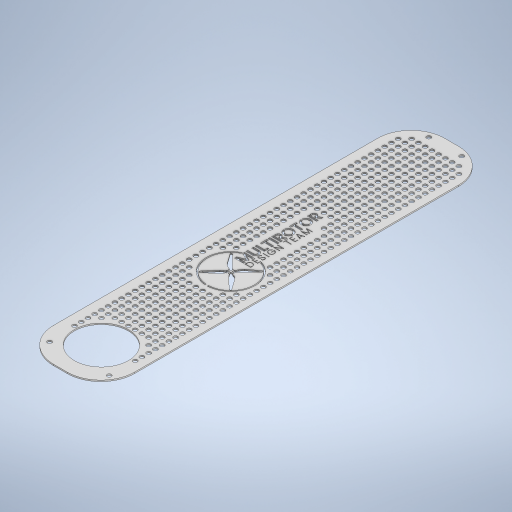
# Autodesk Inventor part: Ground station cover II
Saved by Autodesk Inventor 2023 (Build 270158000, 158)
## iProperties
Created: 2023-04-06
Part Number: Ground station cover II
Material: Generic
Document SubType Name: Modeling
Designer: mikep
Density: 1 g/cm^3
Appearance: Default
Author: mikep
Autodesk Inventor part; units mm, degrees
ref_plane "YZ Plane" through (0, 0, 0) normal (1, 0, 0) x (0, 1, 0)
ref_plane "XZ Plane" through (0, 0, 0) normal (0, 1, 0) x (-1, 0, 0)
ref_plane "XY Plane" through (0, 0, 0) normal (0, 0, 1) x (1, 0, 0)
sketch "Sketch1" plane through (0, 0, 0) normal (0, 1, 0) x (-1, 0, 0)
  line L0 (76.2, 0) -> (76.2, -342.9)
  line L1 (76.2, -342.9) -> (0, -342.9)
  line L2 (0, -342.9) -> (0, 0)
  line L3 (76.2, 0) -> (76.2, 25.4266)
  line L4 (76.2, 25.4266) -> (0, 25.4266)
  line L5 (0, 25.4266) -> (0, 0)
  constraints: 12 end point, 1 collinear, 1 parallel, 1 perpendicular, 1 vertical
extrude "Extrusion1" add sketch "Sketch1" along normal blind 1.27
sketch "Sketch4" plane through (0, 1.27, 0) normal (0, 1, 0) x (1, 0, 0)
  line L0 (-80.9566, 247.2278) -> (206.594, 247.2278)
  line L1 (206.594, 247.2278) -> (206.594, 87.4775)
  line L2 (206.594, 87.4775) -> (-80.9566, 87.4775)
  line L3 (-80.9566, 87.4775) -> (-80.9566, 247.2278)
  line L4 (-41.6156, 195.7662) -> (-41.6156, 195.7662)
  line L5 (-41.6156, 189.984) -> (-41.6156, 189.984)
  line L6 (-45.9155, 181.21) -> (-37.2389, 181.21)
  line L7 (-37.2389, 181.21) -> (-37.2389, 182.9014)
  line L8 (-37.2389, 182.9014) -> (-40.6526, 182.9014)
  line L9 (-40.6526, 183.7206) -> (-37.2389, 185.6718)
  line L10 (-37.2389, 185.6718) -> (-37.2389, 187.5783)
  line L11 (-37.2389, 187.5783) -> (-40.7469, 185.5482)
  arc A0 (-40.7469, 185.5482) -> (-45.5892, 186.0256) centre (-43.2468, 184.9881) ccw
  arc A1 (-45.5892, 186.0256) -> (-45.9155, 184.4827) centre (-42.1055, 184.4827) ccw
  line L12 (-44.4996, 182.9014) -> (-41.931, 182.9014)
  line L13 (-41.931, 183.7206) -> (-41.931, 184.5099)
  line L14 (-44.4996, 183.7206) -> (-44.4996, 184.5099)
  arc A2 (-41.931, 184.5099) -> (-44.4996, 184.5099) centre (-43.2153, 184.5099) ccw
  line L15 (-44.4996, 182.9014) -> (-45.9155, 182.9014)
  line L16 (-41.931, 182.9014) -> (-40.6526, 182.9014)
  line L17 (-40.6526, 183.7206) -> (-41.931, 183.7206)
  line L18 (-44.4996, 183.7206) -> (-45.9155, 183.7206)
  line L19 (-45.9155, 181.21) -> (-45.9155, 182.9014)
  line L20 (-45.9155, 183.7206) -> (-45.9155, 184.4827)
  line L21 (-44.4639, 192.4254) -> (-46.0536, 192.4254)
  line L22 (-44.4639, 193.4122) -> (-46.0419, 193.4122)
  line L23 (-38.7674, 192.4254) -> (-37.1776, 192.4254)
  line L24 (-37.1894, 193.4122) -> (-38.7674, 193.4122)
  arc A3 (-41.6156, 189.984) -> (-38.7674, 192.4254) centre (-41.6156, 192.8661) ccw
  arc A4 (-38.7674, 193.4122) -> (-41.6156, 195.7662) centre (-41.6156, 192.8661) ccw
  arc A5 (-37.1894, 193.4122) -> (-46.0419, 193.4122) centre (-41.6156, 192.8661) ccw
  arc A6 (-46.0536, 192.4254) -> (-37.1776, 192.4254) centre (-41.6156, 192.8661) ccw
  arc A7 (-44.4639, 192.4254) -> (-41.6156, 189.984) centre (-41.6156, 192.8661) ccw
  arc A8 (-41.6156, 195.7662) -> (-44.4639, 193.4122) centre (-41.6156, 192.8661) ccw
  point P0 (0, 0)
  point P1 (-41.6156, 195.7662)
  constraints: 42 end point, 18 point on circle, 9 centre point, 9 tangent, 8 perpendicular, 6 point on line, 4 horizontal, 3 concentric, 3 vertical, 2 parallel, 2 other
sketch "Sketch5" plane through (0, 1.27, 0) normal (0, 1, 0) x (1, 0, 0)
  line L0 (-45.9155, 146.2008) -> (-37.3157, 146.2008)
  line L1 (-37.3157, 146.2008) -> (-37.3157, 147.9554)
  line L2 (-37.3157, 147.9554) -> (-42.8395, 147.9554)
  line L3 (-42.8395, 147.9554) -> (-37.3157, 150.2733)
  line L4 (-37.3157, 150.2733) -> (-37.3157, 151.6596)
  line L5 (-37.3157, 151.6596) -> (-42.8395, 153.9342)
  line L6 (-42.8395, 153.9342) -> (-37.3157, 153.9342)
  line L7 (-37.3157, 153.9342) -> (-37.3157, 155.6671)
  line L8 (-37.3157, 155.6671) -> (-45.9155, 155.6671)
  line L9 (-45.9155, 155.6671) -> (-45.9155, 153.7609)
  line L10 (-45.9155, 153.7609) -> (-39.5036, 150.9664)
  line L11 (-39.5036, 150.9664) -> (-45.9155, 148.2759)
  line L12 (-45.9155, 148.2759) -> (-45.9155, 146.2008)
  line L13 (-45.9155, 157.0446) -> (-40.7133, 157.0446)
  arc A0 (-40.7133, 157.0446) -> (-40.7133, 164.1529) centre (-40.7133, 160.5987) ccw
  line L14 (-40.7133, 164.1529) -> (-45.9155, 164.1529)
  line L15 (-45.9155, 164.1529) -> (-45.9155, 162.4414)
  line L16 (-45.9155, 162.4414) -> (-40.4687, 162.4414)
  arc A1 (-40.4687, 158.8303) -> (-40.4687, 162.4414) centre (-40.4687, 160.6359) ccw
  line L17 (-40.4687, 158.8303) -> (-45.9155, 158.8303)
  line L18 (-45.9155, 158.8303) -> (-45.9155, 157.0446)
  line L19 (-45.9155, 165.5688) -> (-37.3157, 165.5688)
  line L20 (-37.3157, 165.5688) -> (-37.3157, 170.1637)
  line L21 (-37.3157, 170.1637) -> (-38.7004, 170.1637)
  line L22 (-41.8983, 212.0398) -> (-41.3637, 212.0398)
  line L23 (-41.3637, 206.7132) -> (-41.8983, 206.7132)
  line L24 (-45.9155, 197.9622) -> (-45.9155, 204.2278)
  line L25 (-45.9155, 204.2278) -> (-44.5825, 204.2278)
  line L26 (-44.5825, 204.2278) -> (-44.5825, 202.014)
  line L27 (-44.5825, 202.014) -> (-37.2602, 202.014)
  line L28 (-37.2602, 202.014) -> (-37.2602, 200.2387)
  line L29 (-37.2602, 200.2387) -> (-44.5825, 200.2387)
  line L30 (-44.5825, 200.2387) -> (-44.5825, 197.9622)
  line L31 (-44.5825, 197.9622) -> (-45.9155, 197.9622)
  line L32 (-45.9155, 165.5688) -> (-45.9155, 167.334)
  line L33 (-45.9155, 167.334) -> (-38.7004, 167.334)
  line L34 (-38.7004, 167.334) -> (-38.7004, 170.1637)
  line L35 (-45.9155, 170.5777) -> (-45.9155, 176.9008)
  line L36 (-45.9155, 176.9008) -> (-44.5825, 176.9008)
  line L37 (-44.5825, 176.9008) -> (-44.5825, 174.6319)
  line L38 (-44.5825, 174.6319) -> (-37.2602, 174.6319)
  line L39 (-37.2602, 174.6319) -> (-37.2602, 172.8987)
  line L40 (-37.2602, 172.8987) -> (-44.5825, 172.8987)
  line L41 (-44.5825, 172.8987) -> (-44.5825, 170.5777)
  line L42 (-44.5825, 170.5777) -> (-45.9155, 170.5777)
  line L43 (-45.9155, 177.9182) -> (-37.2602, 177.9182)
  line L44 (-37.2602, 177.9182) -> (-37.2602, 179.7056)
  line L45 (-37.2602, 179.7056) -> (-45.9155, 179.7056)
  line L46 (-45.9155, 179.7056) -> (-45.9155, 177.9182)
  line L47 (-45.9123, 214.8446) -> (-37.2357, 214.8446)
  line L48 (-37.2357, 214.8446) -> (-37.2357, 216.536)
  line L49 (-37.2357, 216.536) -> (-40.6494, 216.536)
  line L50 (-40.6494, 217.3525) -> (-40.6494, 217.3552)
  line L51 (-40.6494, 217.3552) -> (-37.2357, 219.3064)
  line L52 (-37.2357, 219.3064) -> (-37.2357, 221.2129)
  line L53 (-37.2357, 221.2129) -> (-40.7436, 219.1829)
  arc A2 (-40.7436, 219.1829) -> (-45.5859, 219.6602) centre (-43.2435, 218.6227) ccw
  arc A3 (-45.5859, 219.6602) -> (-45.9123, 218.1173) centre (-42.1022, 218.1173) ccw
  line L54 (-44.4963, 216.536) -> (-41.9277, 216.536)
  line L55 (-41.9277, 217.3525) -> (-41.9277, 218.1446)
  line L56 (-44.4963, 217.1678) -> (-44.4963, 218.1446)
  arc A4 (-41.9277, 218.1446) -> (-44.4963, 218.1446) centre (-43.212, 218.1446) ccw
  line L57 (-36.1361, 146.2008) -> (-30.6109, 146.2008)
  arc A5 (-30.6109, 148.0046) -> (-36.1361, 148.0046) centre (-33.3735, 148.0046) ccw
  line L58 (-35.7015, 146.7358) -> (-31.0051, 146.7358)
  arc A6 (-31.0051, 147.9604) -> (-35.7015, 147.9604) centre (-33.3533, 147.9604) ccw
  line L59 (-36.2043, 155.6671) -> (-36.2043, 152.7969)
  line L60 (-36.2043, 152.7969) -> (-30.6109, 152.7969)
  line L61 (-30.6109, 152.7969) -> (-30.6109, 155.6671)
  line L62 (-30.6109, 155.6671) -> (-31.0051, 155.6671)
  line L63 (-31.0051, 155.6671) -> (-31.0051, 153.3096)
  line L64 (-31.0051, 153.3096) -> (-33.1818, 153.3096)
  line L65 (-33.1818, 153.3096) -> (-33.1818, 155.4455)
  line L66 (-33.1818, 155.4455) -> (-33.6491, 155.4455)
  line L67 (-33.6491, 155.4455) -> (-33.6491, 153.3096)
  line L68 (-33.6491, 153.3096) -> (-35.7015, 153.3096)
  line L69 (-35.7015, 153.3096) -> (-35.7015, 155.6671)
  line L70 (-35.7015, 155.6671) -> (-36.2043, 155.6671)
  arc A7 (-34.9009, 160.6161) -> (-34.4089, 158.0946) centre (-34.5795, 159.3701) ccw
  arc A8 (-34.9009, 161.1543) -> (-34.4866, 157.5247) centre (-34.573, 159.3533) ccw
  arc A9 (-34.4866, 157.5247) -> (-33.5978, 158.2134) centre (-34.5328, 158.5023) ccw
  arc A10 (-34.4089, 158.0946) -> (-33.9237, 158.5805) centre (-34.6273, 158.7979) ccw
  line L71 (-33.9237, 158.5805) -> (-33.4038, 160.2634)
  line L72 (-33.5978, 158.2134) -> (-33.0272, 160.0606)
  arc A11 (-31.1407, 160.1849) -> (-33.0272, 160.0606) centre (-32.0602, 159.7619) ccw
  arc A12 (-30.6757, 160.2518) -> (-33.4038, 160.2634) centre (-32.0415, 159.8426) ccw
  arc A13 (-31.1407, 158.6615) -> (-31.1407, 160.1849) centre (-32.7961, 159.4232) ccw
  arc A14 (-32.0271, 158.1529) -> (-31.1407, 158.6615) centre (-31.9411, 159.0298) ccw
  arc A15 (-30.8736, 158.0903) -> (-30.6757, 160.2518) centre (-33.4619, 159.417) ccw
  arc A16 (-32.0271, 157.6019) -> (-30.8736, 158.0903) centre (-31.7422, 158.5356) ccw
  line L73 (-32.0271, 157.6019) -> (-32.0271, 158.1529)
  line L74 (-36.2043, 163.2972) -> (-30.5655, 163.2972)
  line L75 (-30.5655, 163.2972) -> (-30.5655, 163.8154)
  line L76 (-30.5655, 163.8154) -> (-36.2043, 163.8154)
  line L77 (-36.2043, 163.8154) -> (-36.2043, 163.2972)
  line L78 (-34.6103, 170.4888) -> (-34.6103, 171.0587)
  arc A17 (-34.6103, 170.4888) -> (-34.6103, 166.6847) centre (-33.6858, 168.5867) ccw
  arc A18 (-34.6103, 171.0587) -> (-34.6103, 166.0747) centre (-33.5706, 168.5667) ccw
  arc A19 (-34.6103, 166.6847) -> (-32.1267, 166.6847) centre (-33.3685, 169.1007) ccw
  arc A20 (-34.6103, 166.0747) -> (-32.1447, 166.0853) centre (-33.39, 168.9994) ccw
  arc A21 (-32.1267, 166.6847) -> (-32.1267, 170.4888) centre (-33.1517, 168.5867) ccw
  arc A22 (-32.1447, 166.0853) -> (-32.1447, 171.1174) centre (-33.3594, 168.6014) ccw
  line L79 (-32.1447, 166.0853) -> (-32.1447, 171.1174) construction
  line L80 (-32.1447, 166.0853) -> (-27.1125, 166.0853) construction
  arc A23 (-32.1267, 170.4888) -> (-33.0883, 170.6871) centre (-32.9388, 168.9819) ccw
  arc A24 (-32.1447, 171.1174) -> (-32.9486, 171.3013) centre (-32.9486, 169.4522) ccw
  line L81 (-33.0883, 170.6871) -> (-33.0883, 168.3488)
  line L82 (-33.0883, 168.3488) -> (-33.5713, 168.3488)
  line L83 (-33.5713, 168.3488) -> (-33.5713, 171.3013)
  line L84 (-33.5713, 171.3013) -> (-32.9486, 171.3013)
  line L85 (-30.5851, 173.2809) -> (-36.2043, 173.2809)
  line L86 (-36.2043, 173.2809) -> (-36.2043, 173.8147)
  line L87 (-36.2043, 173.8147) -> (-31.5027, 176.9008)
  line L88 (-31.5027, 176.9008) -> (-36.2043, 176.9008)
  line L89 (-36.2043, 176.9008) -> (-36.2043, 177.5031)
  line L90 (-36.2043, 177.5031) -> (-30.5851, 177.5031)
  line L91 (-30.5851, 177.5031) -> (-30.5851, 176.9008)
  line L92 (-30.5851, 176.9008) -> (-35.2868, 173.8147)
  line L93 (-35.2868, 173.8147) -> (-30.5851, 173.8147)
  line L94 (-30.5851, 173.8147) -> (-30.5851, 173.2809)
  line L95 (-36.2043, 182.4231) -> (-36.2043, 186.111)
  line L96 (-36.2043, 186.111) -> (-35.7015, 186.111)
  line L97 (-35.7015, 186.111) -> (-35.7015, 184.5808)
  line L98 (-35.7015, 184.5808) -> (-30.5851, 184.5808)
  line L99 (-30.5851, 184.5808) -> (-30.5851, 184.0076)
  line L100 (-30.5851, 184.0076) -> (-35.7015, 184.0076)
  line L101 (-35.7015, 184.0076) -> (-35.7015, 182.4231)
  line L102 (-35.7015, 182.4231) -> (-36.2043, 182.4231)
  line L103 (-36.2043, 187.9758) -> (-36.2043, 190.8754)
  line L104 (-36.2043, 190.8754) -> (-35.7464, 190.8754)
  line L105 (-35.7464, 190.8754) -> (-35.7464, 188.5016)
  line L106 (-35.7464, 188.5016) -> (-33.6172, 188.5016)
  line L107 (-33.6172, 188.5016) -> (-33.6172, 190.6504)
  line L108 (-33.6172, 190.6504) -> (-33.1818, 190.6504)
  line L109 (-33.1818, 190.6504) -> (-33.2075, 188.4955)
  line L110 (-33.2075, 188.4955) -> (-31.0568, 188.4699)
  line L111 (-31.0568, 188.4699) -> (-31.0286, 190.8383)
  line L112 (-31.0286, 190.8383) -> (-30.5851, 190.833)
  line L113 (-30.5851, 190.833) -> (-30.6192, 187.9758)
  line L114 (-30.6192, 187.9758) -> (-36.2043, 187.9758)
  line L115 (-36.0981, 194.6003) -> (-36.0981, 195.1894)
  line L116 (-30.5379, 197.1874) -> (-30.5379, 196.6332)
  line L117 (-30.5379, 196.6332) -> (-31.8644, 196.1565)
  line L118 (-31.8644, 193.5948) -> (-30.5379, 193.1069)
  line L119 (-30.5379, 193.1069) -> (-30.5379, 192.5551)
  line L120 (-30.6192, 199.1004) -> (-36.0958, 199.1004)
  line L121 (-36.0958, 199.1004) -> (-36.0958, 199.6747)
  line L122 (-36.0958, 199.6747) -> (-31.3653, 201.8102)
  line L123 (-31.3653, 201.8102) -> (-36.0958, 203.9571)
  line L124 (-36.0958, 203.9571) -> (-36.0958, 204.5166)
  line L125 (-36.0958, 204.5166) -> (-30.6192, 204.5166)
  line L126 (-30.6192, 204.5166) -> (-30.6192, 204.0028)
  line L127 (-30.6192, 204.0028) -> (-35.0644, 204.0028)
  line L128 (-35.0644, 204.0028) -> (-30.6192, 201.9853)
  line L129 (-30.6192, 201.9853) -> (-30.6192, 201.6879)
  line L130 (-30.6192, 201.6879) -> (-34.9638, 199.6747)
  line L131 (-34.9638, 199.6747) -> (-30.6192, 199.6747)
  line L132 (-30.6192, 199.6747) -> (-30.6192, 199.1004)
  line L133 (-29.8128, 154.4415) -> (-29.8128, 155.5845)
  line L134 (-46.6367, 153.1669) -> (-46.6367, 154.3802)
  arc A25 (-37.3019, 131.531) -> (-38.3544, 129.2661) centre (-33.6753, 128.4687) ccw
  arc A26 (-39.931, 126.4634) -> (-38.3544, 129.2661) centre (-43.0594, 130.0679) ccw
  line L135 (-39.931, 126.4634) -> (-51.2653, 117.782)
  arc A27 (-51.6556, 119.3522) -> (-51.2653, 117.782) centre (-50.6262, 118.7744) ccw
  arc A28 (-50.7672, 120.6762) -> (-51.6556, 119.3522) centre (-42.9118, 114.4448) ccw
  line L136 (-50.7672, 120.6762) -> (-43.0339, 129.1527)
  arc A29 (-40.9214, 131.0009) -> (-43.0339, 129.1527) centre (-33.7965, 120.7253) ccw
  arc A30 (-40.9214, 131.0009) -> (-38.9896, 132.5554) centre (-50.8331, 145.2957) ccw
  arc A31 (-35.5046, 136.0705) -> (-35.3221, 136.4134) centre (-35.9841, 136.5458) ccw
  arc A32 (-34.5137, 138.6581) -> (-35.3221, 136.4134) centre (-27.4046, 134.8301) ccw
  arc A33 (-31.9411, 142.1183) -> (-34.5137, 138.6581) centre (-21.4115, 131.6031) ccw
  line L137 (-31.9411, 142.1183) -> (-22.0341, 149.4341)
  arc A34 (-21.5184, 147.9604) -> (-22.0341, 149.4341) centre (-22.6014, 148.4085) ccw
  arc A35 (-22.1375, 147.004) -> (-21.5184, 147.9604) centre (-24.4242, 149.1628) ccw
  line L138 (-22.1375, 147.004) -> (-32.1455, 136.4032)
  arc A36 (-32.6979, 135.9774) -> (-32.1455, 136.4032) centre (-33.7632, 137.9304) ccw
  arc A37 (-32.6979, 135.9774) -> (-34.232, 134.8088) centre (-29.6411, 130.3732) ccw
  arc A38 (-34.7465, 133.0816) -> (-31.7342, 131.6031) centre (-30.9458, 137.0173) ccw
  arc A39 (-30.3913, 131.0009) -> (-31.7342, 131.6031) centre (-32.1221, 128.9395) ccw
  arc A40 (-27.8576, 128.297) -> (-30.3913, 131.0009) centre (-40.3881, 119.0944) ccw
  line L139 (-27.8939, 128.3463) -> (-21.0506, 118.672)
  arc A41 (-22.9089, 118.3552) -> (-21.0506, 118.672) centre (-22.1356, 119.4277) ccw
  arc A42 (-24.0971, 119.3522) -> (-22.9089, 118.3552) centre (-16.7176, 126.9409) ccw
  line L140 (-24.0971, 119.3522) -> (-33.3887, 128.4687)
  arc A43 (-35.1974, 130.7141) -> (-33.3887, 128.4687) centre (-24.7254, 137.2984) ccw
  line L141 (-35.1974, 130.7141) -> (-36.0908, 131.7691)
  line L142 (-38.4118, 134.2018) -> (-38.9896, 134.8301)
  arc A44 (-37.8105, 136.1187) -> (-38.8384, 137.4254) centre (-53.9232, 124.5022) ccw
  line L143 (-38.8384, 137.4254) -> (-49.6093, 148.2759)
  arc A45 (-49.6093, 148.2759) -> (-50.5164, 148.9551) centre (-52.3671, 145.5384) ccw
  arc A46 (-50.5164, 148.9551) -> (-52.0337, 148.4508) centre (-50.9672, 147.7767) ccw
  line L144 (-52.0337, 148.4508) -> (-45.145, 138.6581)
  arc A47 (-45.145, 138.6581) -> (-42.0297, 136.1187) centre (-39.0672, 142.9336) ccw
  arc A48 (-42.0297, 136.1187) -> (-38.9896, 134.8301) centre (29.7401, 301.2179) ccw
  line L145 (-35.7015, 147.1027) -> (-36.1361, 147.1027)
  line L146 (-35.7015, 147.5439) -> (-36.1361, 147.5439)
  line L147 (-36.1361, 146.2008) -> (-36.1361, 147.1027)
  line L148 (-36.1361, 147.5439) -> (-36.1361, 148.0046)
  line L149 (-35.7015, 146.7358) -> (-35.7015, 147.1027)
  line L150 (-35.7015, 147.5439) -> (-35.7015, 147.9604)
  line L151 (-31.0051, 147.1027) -> (-30.6109, 147.1027)
  line L152 (-31.0051, 147.4539) -> (-30.6109, 147.4539)
  line L153 (-31.0051, 146.7358) -> (-31.0051, 147.1027)
  line L154 (-31.0051, 147.4539) -> (-31.0051, 147.9604)
  line L155 (-30.6109, 146.2008) -> (-30.6109, 147.1027)
  line L156 (-30.6109, 147.4539) -> (-30.6109, 148.0046)
  line L157 (-44.4963, 208.79) -> (-46.0225, 208.79)
  line L158 (-44.4963, 209.963) -> (-46.0085, 209.963)
  line L159 (-48.0365, 209.3765) -> (-35.9188, 209.3765)
  arc A49 (-41.8983, 212.0398) -> (-44.4963, 209.963) centre (-41.8983, 209.3765) ccw
  arc A50 (-44.4963, 208.79) -> (-41.8983, 206.7132) centre (-41.8983, 209.3765) ccw
  line L160 (-38.7658, 208.79) -> (-37.167, 208.79)
  line L161 (-38.7658, 209.963) -> (-37.181, 209.963)
  arc A51 (-41.3637, 206.7132) -> (-38.7658, 208.79) centre (-41.3637, 209.3765) ccw
  arc A52 (-38.7658, 209.963) -> (-41.3637, 212.0398) centre (-41.3637, 209.3765) ccw
  arc A53 (-46.0225, 208.79) -> (-37.167, 208.79) centre (-41.5947, 209.3239) ccw
  arc A54 (-37.181, 209.963) -> (-46.0085, 209.963) centre (-41.5947, 209.3239) ccw
  line L162 (-44.4963, 216.536) -> (-45.9123, 216.536)
  line L163 (-44.4963, 217.1678) -> (-45.9123, 217.1678)
  line L164 (-45.9123, 214.8446) -> (-45.9123, 216.536)
  line L165 (-45.9123, 217.1678) -> (-45.9123, 218.1173)
  line L166 (-41.9277, 216.536) -> (-40.6494, 216.536)
  line L167 (-41.9277, 217.3525) -> (-40.6494, 217.3525)
  line L168 (-32.3182, 193.7321) -> (-32.3182, 195.0363)
  line L169 (-31.8644, 195.0363) -> (-31.8644, 193.5948)
  line L170 (-30.5379, 192.5551) -> (-33.949, 193.8098)
  line L171 (-33.7774, 194.2773) -> (-32.3182, 193.7321)
  line L172 (-34.1396, 195.339) -> (-34.1398, 195.3396)
  line L173 (-36.0981, 195.1894) -> (-34.1433, 195.8918)
  line L174 (-34.1433, 195.8918) -> (-30.5379, 197.1874)
  line L175 (-34.275, 195.2866) -> (-35.3601, 194.8616)
  line L176 (-34.9009, 160.6161) -> (-34.9009, 161.1543)
  line L177 (-36.6964, 133.6313) -> (-36.6964, 157.6019) construction
  line L178 (-36.6964, 157.6019) -> (-36.6964, 133.6313) construction
  line L179 (-36.6964, 133.6313) -> (-36.6964, 133.0816) construction
  line L180 (-37.9664, 110.6593) -> (-37.9664, 111.7491)
  line L181 (-35.911, 110.6377) -> (-35.911, 111.7263)
  arc A55 (-46.6367, 154.3802) -> (-37.9664, 110.6593) centre (-36.6964, 133.6313) ccw
  arc A56 (-35.911, 110.6377) -> (-29.8128, 155.5845) centre (-36.6964, 133.6313) ccw
  arc A57 (-46.6367, 153.1669) -> (-37.9664, 111.7491) centre (-36.6964, 133.6313) ccw
  arc A58 (-35.911, 111.7263) -> (-29.8128, 154.4415) centre (-36.6964, 133.6313) ccw
  line L182 (-35.1318, 194.2449) -> (-34.4319, 194.519)
  line L183 (-36.0583, 194.5856) -> (-35.357, 194.8604)
  line L184 (-32.3182, 195.4099) -> (-31.8644, 195.5964)
  line L185 (-32.3182, 195.0363) -> (-32.3182, 195.4099)
  line L186 (-32.3182, 196.0509) -> (-32.3182, 196.0533)
  line L187 (-31.8644, 195.5964) -> (-31.8644, 195.0363)
  line L188 (-35.3601, 194.8616) -> (-35.357, 194.8604)
  line L189 (-34.4321, 194.519) -> (-33.7774, 194.2773)
  line L190 (-33.949, 193.8098) -> (-35.1318, 194.2449)
  line L191 (-36.0583, 194.5856) -> (-36.0981, 194.6003)
  line L192 (-31.8644, 196.1565) -> (-34.275, 195.2866)
  line L193 (-34.232, 134.8088) -> (-34.8022, 134.2018)
  arc A59 (-37.8652, 130.6992) -> (-37.3019, 130.5335) centre (-36.6964, 133.6313) ccw
  arc A60 (-36.0908, 130.5335) -> (-35.2794, 130.8108) centre (-36.6964, 133.6313) ccw
  arc A61 (-39.5166, 135.0488) -> (-39.8009, 134.2018) centre (-36.6964, 133.6313) ccw
  arc A62 (-39.8046, 133.0816) -> (-39.4702, 132.125) centre (-36.6964, 133.6313) ccw
  arc A63 (-35.3111, 136.4675) -> (-36.0908, 136.7292) centre (-36.6964, 133.6313) ccw
  arc A64 (-37.3019, 136.7292) -> (-38.0716, 136.4725) centre (-36.6964, 133.6313) ccw
  arc A65 (-33.8094, 132.3552) -> (-33.5882, 133.0816) centre (-36.6964, 133.6313) ccw
  arc A66 (-33.5919, 134.2018) -> (-33.9119, 135.1179) centre (-36.6964, 133.6313) ccw
  line L194 (-38.4679, 133.0816) -> (-38.9896, 132.5554)
  line L195 (-37.3019, 130.5335) -> (-37.3019, 133.0816)
  line L196 (-37.3019, 134.2018) -> (-37.3019, 136.7292)
  line L197 (-36.0908, 136.7292) -> (-36.0908, 134.2018)
  line L198 (-36.0908, 133.0816) -> (-36.0908, 130.5335)
  line L199 (-39.8046, 133.0816) -> (-37.3019, 133.0816)
  line L200 (-36.0908, 133.0816) -> (-33.5882, 133.0816)
  line L201 (-33.5919, 134.2018) -> (-36.0908, 134.2018)
  line L202 (-37.3019, 134.2018) -> (-39.8009, 134.2018)
  line L203 (-37.8105, 136.1187) -> (-37.3019, 135.6145)
  line L204 (-35.5046, 136.0705) -> (-36.0908, 135.4792)
  point P0 (0, 0)
  point P1 (-45.2594, 208.79)
  point P2 (-37.9664, 208.79)
  point P3 (-31.8644, 194.7801)
  point P4 (-34.275, 193.9297)
  point P5 (-34.1033, 194.3976)
  point P6 (-32.0913, 194.7801)
  point P7 (-34.1879, 194.1658)
  point P8 (-33.862, 194.0455)
  point P9 (-35.911, 111.182)
  point P10 (-37.9664, 111.2042)
  point P11 (-33.6491, 195.5319)
  point P12 (-41.2885, 217.3525)
  dimension "d64" = 0.5865
  dimension "d65" = 0.5865
  dimension "d66" = 0.5865
  dimension "d118" = 1.27
  dimension "d119" = 2.0554
  dimension "d136" = 0.1846
  constraints: 410 end point, 142 point on circle, 86 perpendicular, 67 centre point, 54 tangent, 51 point on line, 31 parallel, 23 vertical, 21 horizontal, 5 midpoint, 2 coincident, 2 collinear
  measures "d64" distance from line of L159 point (-45.259, 208.79)
  measures "d65" distance from line of point (-37.966, 208.79) L159
  measures "d66" distance between parallel lines of L159 L161
  measures "d118" distance between parallel lines of L179 L180
  measures "d119" horizontal distance of point (-35.911, 111.182) point (-37.966, 111.204)
  measures "d136" distance from line of point (-41.289, 217.352) L163
extrude "Extrusion4" cut sketch "Sketch5" against normal blind 12.7
extrude "Extrusion5" cut sketch "Sketch4" against normal blind 12.7 contours L19 L15 L12 L16 L8 L7 L6 | L17 L13 A2 L14 L18 L20 A1 A0 L11 L10 L9 | A7 A3 L23 A6 L21 | L22 A5 L24 A4 A8
sketch "Sketch6" plane through (0, 1.27, 0) normal (0, 1, 0) x (1, 0, 0)
  line L0 (-76.2, 0) -> (0, 0) projected
  circle A0 centre (-37.6477, 12.7) radius 25.4
  dimension "d84" = 50.8
  constraints: 1 centre point
  measures "d84" diameter of A0
extrude "Extrusion6" cut sketch "Sketch6" against normal blind 12.7
sketch "Sketch7" plane through (0, 1.27, 0) normal (0, 1, 0) x (1, 0, 0)
  line L0 (0, 342.9) -> (-76.2, 342.9) projected
  line L1 (-76.2, -25.4266) -> (0, -25.4266) projected
  point P0 (0, 0)
  point P1 (-64.6374, -9.0958)
  point P2 (-21.9942, 336.3525)
  point P3 (-9.1559, -8.4866)
  point P4 (-52.902, 336.2531)
hole "Hole1" at (-64.6374, 1.27, 9.0958) at (-21.9942, 1.27, -336.3525) at (-52.902, 1.27, -336.2531) at (-9.1559, 1.27, 8.4866) direction (0, -1, 0) diameter 4 depth 19.05 tip angle 118
sketch "Sketch8" plane through (0, 1.27, 0) normal (0, 1, 0) x (1, 0, 0)
  line L0 (-68.6346, 12.7) -> (-3.5822, 12.7) construction
  line L1 (-66.342, 330.2) -> (-9.6002, 330.2) construction
  line L2 (0, 342.9) -> (-76.2, 342.9) projected
  line L3 (-68.6346, 12.7) -> (-68.6346, 330.2) construction
  point P0 (0, 0)
  point P1 (-66.0005, 15.7195)
  point P2 (-66.0005, 22.0695)
  point P3 (-66.0005, 28.4195)
  point P4 (-66.0005, 34.7695)
  point P5 (-66.0005, 41.1195)
  point P6 (-66.0005, 47.4695)
  point P7 (-66.0005, 53.8195)
  point P8 (-66.0005, 60.1695)
  point P9 (-66.0005, 66.5195)
  point P10 (-66.0005, 72.8695)
  point P11 (-66.0005, 79.2195)
  point P12 (-66.0005, 85.5695)
  point P13 (-66.0005, 91.9195)
  point P14 (-66.0005, 98.2695)
  point P15 (-66.0005, 104.6195)
  point P16 (-66.0005, 110.9695)
  point P17 (-66.0005, 117.3195)
  point P18 (-66.0005, 123.6695)
  point P19 (-66.0005, 130.0195)
  point P20 (-66.0005, 136.3695)
  point P21 (-66.0005, 142.7195)
  point P22 (-66.0005, 149.0695)
  point P23 (-66.0005, 155.4195)
  point P24 (-66.0005, 161.7695)
  point P25 (-66.0005, 168.1195)
  point P26 (-66.0005, 174.4695)
  point P27 (-66.0005, 180.8195)
  point P28 (-66.0005, 187.1695)
  point P29 (-66.0005, 193.5195)
  point P30 (-66.0005, 199.8695)
  point P31 (-66.0005, 206.2195)
  point P32 (-66.0005, 212.5695)
  point P33 (-66.0005, 218.9195)
  point P34 (-66.0005, 225.2695)
  point P35 (-66.0005, 231.6195)
  point P36 (-66.0005, 237.9695)
  point P37 (-66.0005, 244.3195)
  point P38 (-66.0005, 250.6695)
  point P39 (-66.0005, 257.0195)
  point P40 (-66.0005, 263.3695)
  point P41 (-66.0005, 269.7195)
  point P42 (-66.0005, 276.0695)
  point P43 (-66.0005, 282.4195)
  point P44 (-66.0005, 288.7695)
  point P45 (-66.0005, 295.1195)
  point P46 (-66.0005, 301.4695)
  point P47 (-66.0005, 307.8195)
  point P48 (-66.0005, 314.1695)
  point P49 (-66.0005, 320.5195)
  point P50 (-59.6505, 15.7195)
  point P51 (-59.6505, 22.0695)
  point P52 (-59.6505, 28.4195)
  point P53 (-59.6505, 34.7695)
  point P54 (-59.6505, 41.1195)
  point P55 (-59.6505, 47.4695)
  point P56 (-59.6505, 53.8195)
  point P57 (-59.6505, 60.1695)
  point P58 (-59.6505, 66.5195)
  point P59 (-59.6505, 72.8695)
  point P60 (-59.6505, 79.2195)
  point P61 (-59.6505, 85.5695)
  point P62 (-59.6505, 91.9195)
  point P63 (-59.6505, 98.2695)
  point P64 (-59.6505, 104.6195)
  point P65 (-59.6505, 110.9695)
  point P66 (-59.6505, 117.3195)
  point P67 (-59.6505, 123.6695)
  point P68 (-59.6505, 130.0195)
  point P69 (-59.6505, 136.3695)
  point P70 (-59.6505, 142.7195)
  point P71 (-59.6505, 149.0695)
  point P72 (-59.6505, 155.4195)
  point P73 (-59.6505, 161.7695)
  point P74 (-59.6505, 168.1195)
  point P75 (-59.6505, 174.4695)
  point P76 (-59.6505, 180.8195)
  point P77 (-59.6505, 187.1695)
  point P78 (-59.6505, 193.5195)
  point P79 (-59.6505, 199.8695)
  point P80 (-59.6505, 206.2195)
  point P81 (-59.6505, 212.5695)
  point P82 (-59.6505, 218.9195)
  point P83 (-59.6505, 225.2695)
  point P84 (-59.6505, 231.6195)
  point P85 (-59.6505, 237.9695)
  point P86 (-59.6505, 244.3195)
  point P87 (-59.6505, 250.6695)
  point P88 (-59.6505, 257.0195)
  point P89 (-59.6505, 263.3695)
  point P90 (-59.6505, 269.7195)
  point P91 (-59.6505, 276.0695)
  point P92 (-59.6505, 282.4195)
  point P93 (-59.6505, 288.7695)
  point P94 (-59.6505, 295.1195)
  point P95 (-59.6505, 301.4695)
  point P96 (-59.6505, 307.8195)
  point P97 (-59.6505, 314.1695)
  point P98 (-59.6505, 320.5195)
  point P99 (-59.6505, 326.8695)
  point P100 (-53.3005, 15.7195)
  point P101 (-53.3005, 22.0695)
  point P102 (-53.3005, 28.4195)
  point P103 (-53.3005, 34.7695)
  point P104 (-53.3005, 41.1195)
  point P105 (-53.3005, 47.4695)
  point P106 (-53.3005, 53.8195)
  point P107 (-53.3005, 60.1695)
  point P108 (-53.3005, 66.5195)
  point P109 (-53.3005, 72.8695)
  point P110 (-53.3005, 79.2195)
  point P111 (-53.3005, 85.5695)
  point P112 (-53.3005, 91.9195)
  point P113 (-53.3005, 98.2695)
  point P114 (-53.3005, 104.6195)
  point P115 (-53.3005, 110.9695)
  point P116 (-53.3005, 117.3195)
  point P117 (-53.3005, 123.6695)
  point P118 (-53.3005, 130.0195)
  point P119 (-53.3005, 136.3695)
  point P120 (-53.3005, 142.7195)
  point P121 (-53.3005, 149.0695)
  point P122 (-53.3005, 155.4195)
  point P123 (-53.3005, 161.7695)
  point P124 (-53.3005, 168.1195)
  point P125 (-53.3005, 174.4695)
  point P126 (-53.3005, 180.8195)
  point P127 (-53.3005, 187.1695)
  point P128 (-53.3005, 193.5195)
  point P129 (-53.3005, 199.8695)
  point P130 (-53.3005, 206.2195)
  point P131 (-53.3005, 212.5695)
  point P132 (-53.3005, 218.9195)
  point P133 (-53.3005, 225.2695)
  point P134 (-53.3005, 231.6195)
  point P135 (-53.3005, 237.9695)
  point P136 (-53.3005, 244.3195)
  point P137 (-53.3005, 250.6695)
  point P138 (-53.3005, 257.0195)
  point P139 (-53.3005, 263.3695)
  point P140 (-53.3005, 269.7195)
  point P141 (-53.3005, 276.0695)
  point P142 (-53.3005, 282.4195)
  point P143 (-53.3005, 288.7695)
  point P144 (-53.3005, 295.1195)
  point P145 (-53.3005, 301.4695)
  point P146 (-53.3005, 307.8195)
  point P147 (-53.3005, 314.1695)
  point P148 (-53.3005, 320.5195)
  point P149 (-53.3005, 326.8695)
  point P150 (-46.9505, 15.7195)
  point P151 (-46.9505, 22.0695)
  point P152 (-46.9505, 28.4195)
  point P153 (-46.9505, 34.7695)
  point P154 (-46.9505, 41.1195)
  point P155 (-46.9505, 47.4695)
  point P156 (-46.9505, 53.8195)
  point P157 (-46.9505, 60.1695)
  point P158 (-46.9505, 66.5195)
  point P159 (-46.9505, 72.8695)
  point P160 (-46.9505, 79.2195)
  point P161 (-46.9505, 85.5695)
  point P162 (-46.9505, 91.9195)
  point P163 (-46.9505, 98.2695)
  point P164 (-46.9505, 104.6195)
  point P165 (-46.9505, 110.9695)
  point P166 (-46.9505, 117.3195)
  point P167 (-46.9505, 123.6695)
  point P168 (-46.9505, 130.0195)
  point P169 (-46.9505, 136.3695)
  point P170 (-46.9505, 142.7195)
  point P171 (-46.9505, 149.0695)
  point P172 (-46.9505, 155.4195)
  point P173 (-46.9505, 161.7695)
  point P174 (-46.9505, 168.1195)
  point P175 (-46.9505, 174.4695)
  point P176 (-46.9505, 180.8195)
  point P177 (-46.9505, 187.1695)
  point P178 (-46.9505, 193.5195)
  point P179 (-46.9505, 199.8695)
  point P180 (-46.9505, 206.2195)
  point P181 (-46.9505, 212.5695)
  point P182 (-46.9505, 218.9195)
  point P183 (-46.9505, 225.2695)
  point P184 (-46.9505, 231.6195)
  point P185 (-46.9505, 237.9695)
  point P186 (-46.9505, 244.3195)
  point P187 (-46.9505, 250.6695)
  point P188 (-46.9505, 257.0195)
  point P189 (-46.9505, 263.3695)
  point P190 (-46.9505, 269.7195)
  point P191 (-46.9505, 276.0695)
  point P192 (-46.9505, 282.4195)
  point P193 (-46.9505, 288.7695)
  point P194 (-46.9505, 295.1195)
  point P195 (-46.9505, 301.4695)
  point P196 (-46.9505, 307.8195)
  point P197 (-46.9505, 314.1695)
  point P198 (-46.9505, 320.5195)
  point P199 (-46.9505, 326.8695)
  dimension "d99" = 12.7
  dimension "d103" = 6.35
  dimension "d106" = 6.35
  constraints: 6 end point, 3 horizontal, 1 perpendicular, 1 point on line, 1 vertical, 496 other
  measures "d99" distance between parallel lines of L2 L1
  measures "d103" distance of point (-66.001, 15.719) point (-66.001, 22.069)
  measures "d106" distance of point (-66.001, 15.719) point (-59.651, 15.719)
hole "Hole2" at (-66.0005, 1.27, -15.7195) at (-66.0005, 1.27, -22.0695) at (-66.0005, 1.27, -28.4195) at (-66.0005, 1.27, -34.7695) at (-66.0005, 1.27, -41.1195) at (-66.0005, 1.27, -47.4695) at (-66.0005, 1.27, -53.8195) at (-66.0005, 1.27, -60.1695) at (-66.0005, 1.27, -66.5195) at (-66.0005, 1.27, -72.8695) at (-66.0005, 1.27, -79.2195) at (-66.0005, 1.27, -85.5695) at (-66.0005, 1.27, -91.9195) at (-66.0005, 1.27, -98.2695) at (-66.0005, 1.27, -104.6195) at (-66.0005, 1.27, -110.9695) at (-66.0005, 1.27, -117.3195) at (-66.0005, 1.27, -123.6695) at (-66.0005, 1.27, -130.0195) at (-66.0005, 1.27, -136.3695) at (-66.0005, 1.27, -142.7195) at (-66.0005, 1.27, -149.0695) at (-66.0005, 1.27, -155.4195) at (-66.0005, 1.27, -161.7695) at (-66.0005, 1.27, -168.1195) at (-66.0005, 1.27, -174.4695) at (-66.0005, 1.27, -180.8195) at (-66.0005, 1.27, -187.1695) at (-66.0005, 1.27, -193.5195) at (-66.0005, 1.27, -199.8695) at (-66.0005, 1.27, -206.2195) at (-66.0005, 1.27, -212.5695) at (-66.0005, 1.27, -218.9195) at (-66.0005, 1.27, -225.2695) at (-66.0005, 1.27, -231.6195) at (-66.0005, 1.27, -237.9695) at (-66.0005, 1.27, -244.3195) at (-66.0005, 1.27, -250.6695) at (-66.0005, 1.27, -257.0195) at (-66.0005, 1.27, -263.3695) at (-66.0005, 1.27, -269.7195) at (-66.0005, 1.27, -276.0695) at (-66.0005, 1.27, -282.4195) at (-66.0005, 1.27, -288.7695) at (-66.0005, 1.27, -295.1195) at (-66.0005, 1.27, -301.4695) at (-66.0005, 1.27, -307.8195) at (-66.0005, 1.27, -314.1695) at (-66.0005, 1.27, -320.5195) at (-59.6505, 1.27, -34.7695) direction (0, -1, 0) diameter 4 depth 19.05 tip angle 118 and at (-59.6505, 1.27, -41.1195) (-59.6505, 1.27, -47.4695) (-59.6505, 1.27, -53.8195) (-59.6505, 1.27, -60.1695) (-59.6505, 1.27, -66.5195) (-59.6505, 1.27, -72.8695) (-59.6505, 1.27, -79.2195) (-59.6505, 1.27, -85.5695) (-59.6505, 1.27, -91.9195) (-59.6505, 1.27, -98.2695) (-59.6505, 1.27, -104.6195) (-59.6505, 1.27, -110.9695) (-59.6505, 1.27, -117.3195) (-59.6505, 1.27, -149.0695) (-59.6505, 1.27, -155.4195) (-59.6505, 1.27, -161.7695) (-59.6505, 1.27, -168.1195) (-59.6505, 1.27, -174.4695) (-59.6505, 1.27, -180.8195) (-59.6505, 1.27, -187.1695) (-59.6505, 1.27, -193.5195) (-59.6505, 1.27, -199.8695) (-59.6505, 1.27, -206.2195) (-59.6505, 1.27, -212.5695) (-59.6505, 1.27, -218.9195) (-59.6505, 1.27, -225.2695) (-59.6505, 1.27, -231.6195) (-59.6505, 1.27, -237.9695) (-59.6505, 1.27, -244.3195) (-59.6505, 1.27, -250.6695) (-59.6505, 1.27, -257.0195) (-59.6505, 1.27, -263.3695) (-59.6505, 1.27, -269.7195) (-59.6505, 1.27, -276.0695) (-59.6505, 1.27, -282.4195) (-59.6505, 1.27, -288.7695) (-59.6505, 1.27, -295.1195) (-59.6505, 1.27, -301.4695) (-59.6505, 1.27, -307.8195) (-59.6505, 1.27, -314.1695) (-59.6505, 1.27, -320.5195) (-59.6505, 1.27, -326.8695) (-53.3005, 1.27, -41.1195) (-53.3005, 1.27, -47.4695) (-53.3005, 1.27, -53.8195) (-53.3005, 1.27, -60.1695) (-53.3005, 1.27, -66.5195) (-53.3005, 1.27, -72.8695) (-53.3005, 1.27, -79.2195) (-53.3005, 1.27, -85.5695) (-53.3005, 1.27, -91.9195) (-53.3005, 1.27, -98.2695) (-53.3005, 1.27, -104.6195) (-53.3005, 1.27, -110.9695) (-53.3005, 1.27, -155.4195) (-53.3005, 1.27, -161.7695) (-53.3005, 1.27, -168.1195) (-53.3005, 1.27, -174.4695) (-53.3005, 1.27, -180.8195) (-53.3005, 1.27, -187.1695) (-53.3005, 1.27, -193.5195) (-53.3005, 1.27, -199.8695) (-53.3005, 1.27, -206.2195) (-53.3005, 1.27, -212.5695) (-53.3005, 1.27, -218.9195) (-53.3005, 1.27, -225.2695) (-53.3005, 1.27, -231.6195) (-53.3005, 1.27, -237.9695) (-53.3005, 1.27, -244.3195) (-53.3005, 1.27, -250.6695) (-53.3005, 1.27, -257.0195) (-53.3005, 1.27, -263.3695) (-53.3005, 1.27, -269.7195) (-53.3005, 1.27, -276.0695) (-53.3005, 1.27, -282.4195) (-53.3005, 1.27, -288.7695) (-53.3005, 1.27, -295.1195) (-53.3005, 1.27, -301.4695) (-53.3005, 1.27, -307.8195) (-53.3005, 1.27, -314.1695) (-53.3005, 1.27, -320.5195) (-53.3005, 1.27, -326.8695) (-46.9505, 1.27, -41.1195) (-46.9505, 1.27, -47.4695) (-46.9505, 1.27, -53.8195) (-46.9505, 1.27, -60.1695) (-46.9505, 1.27, -66.5195) (-46.9505, 1.27, -72.8695) (-46.9505, 1.27, -79.2195) (-46.9505, 1.27, -85.5695) (-46.9505, 1.27, -91.9195) (-46.9505, 1.27, -98.2695) (-46.9505, 1.27, -104.6195) (-46.9505, 1.27, -225.2695) (-46.9505, 1.27, -231.6195) (-46.9505, 1.27, -237.9695) (-46.9505, 1.27, -244.3195) (-46.9505, 1.27, -250.6695) (-46.9505, 1.27, -257.0195) (-46.9505, 1.27, -263.3695) (-46.9505, 1.27, -269.7195) (-46.9505, 1.27, -276.0695) (-46.9505, 1.27, -282.4195) (-46.9505, 1.27, -288.7695) (-46.9505, 1.27, -295.1195) (-46.9505, 1.27, -301.4695) (-46.9505, 1.27, -307.8195) (-46.9505, 1.27, -314.1695) (-46.9505, 1.27, -320.5195) (-46.9505, 1.27, -326.8695) (-40.6005, 1.27, -41.1195) (-40.6005, 1.27, -47.4695) (-40.6005, 1.27, -53.8195) (-40.6005, 1.27, -60.1695) (-40.6005, 1.27, -66.5195) (-40.6005, 1.27, -72.8695) (-40.6005, 1.27, -79.2195) (-40.6005, 1.27, -85.5695) (-40.6005, 1.27, -91.9195) (-40.6005, 1.27, -98.2695) (-40.6005, 1.27, -104.6195) (-40.6005, 1.27, -225.2695) (-40.6005, 1.27, -231.6195) (-40.6005, 1.27, -237.9695) (-40.6005, 1.27, -244.3195) (-40.6005, 1.27, -250.6695) (-40.6005, 1.27, -257.0195) (-40.6005, 1.27, -263.3695) (-40.6005, 1.27, -269.7195) (-40.6005, 1.27, -276.0695) (-40.6005, 1.27, -282.4195) (-40.6005, 1.27, -288.7695) (-40.6005, 1.27, -295.1195) (-40.6005, 1.27, -301.4695) (-40.6005, 1.27, -307.8195) (-40.6005, 1.27, -314.1695) (-40.6005, 1.27, -320.5195) (-40.6005, 1.27, -326.8695) (-34.2505, 1.27, -41.1195) (-34.2505, 1.27, -47.4695) (-34.2505, 1.27, -53.8195) (-34.2505, 1.27, -60.1695) (-34.2505, 1.27, -66.5195) (-34.2505, 1.27, -72.8695) (-34.2505, 1.27, -79.2195) (-34.2505, 1.27, -85.5695) (-34.2505, 1.27, -91.9195) (-34.2505, 1.27, -98.2695) (-34.2505, 1.27, -104.6195) (-34.2505, 1.27, -225.2695) (-34.2505, 1.27, -231.6195) (-34.2505, 1.27, -237.9695) (-34.2505, 1.27, -244.3195) (-34.2505, 1.27, -250.6695) (-34.2505, 1.27, -257.0195) (-34.2505, 1.27, -263.3695) (-34.2505, 1.27, -269.7195) (-34.2505, 1.27, -276.0695) (-34.2505, 1.27, -282.4195) (-34.2505, 1.27, -288.7695) (-34.2505, 1.27, -295.1195) (-34.2505, 1.27, -301.4695) (-34.2505, 1.27, -307.8195) (-34.2505, 1.27, -314.1695) (-34.2505, 1.27, -320.5195) (-34.2505, 1.27, -326.8695) (-27.9005, 1.27, -41.1195) (-27.9005, 1.27, -47.4695) (-27.9005, 1.27, -53.8195) (-27.9005, 1.27, -60.1695) (-27.9005, 1.27, -66.5195) (-27.9005, 1.27, -72.8695) (-27.9005, 1.27, -79.2195) (-27.9005, 1.27, -85.5695) (-27.9005, 1.27, -91.9195) (-27.9005, 1.27, -98.2695) (-27.9005, 1.27, -104.6195) (-27.9005, 1.27, -212.5695) (-27.9005, 1.27, -218.9195) (-27.9005, 1.27, -225.2695) (-27.9005, 1.27, -231.6195) (-27.9005, 1.27, -237.9695) (-27.9005, 1.27, -244.3195) (-27.9005, 1.27, -250.6695) (-27.9005, 1.27, -257.0195) (-27.9005, 1.27, -263.3695) (-27.9005, 1.27, -269.7195) (-27.9005, 1.27, -276.0695) (-27.9005, 1.27, -282.4195) (-27.9005, 1.27, -288.7695) (-27.9005, 1.27, -295.1195) (-27.9005, 1.27, -301.4695) (-27.9005, 1.27, -307.8195) (-27.9005, 1.27, -314.1695) (-27.9005, 1.27, -320.5195) (-27.9005, 1.27, -326.8695) (-21.5505, 1.27, -41.1195) (-21.5505, 1.27, -47.4695) (-21.5505, 1.27, -53.8195) (-21.5505, 1.27, -60.1695) (-21.5505, 1.27, -66.5195) (-21.5505, 1.27, -72.8695) (-21.5505, 1.27, -79.2195) (-21.5505, 1.27, -85.5695) (-21.5505, 1.27, -91.9195) (-21.5505, 1.27, -98.2695) (-21.5505, 1.27, -104.6195) (-21.5505, 1.27, -110.9695) (-21.5505, 1.27, -155.4195) (-21.5505, 1.27, -161.7695) (-21.5505, 1.27, -168.1195) (-21.5505, 1.27, -174.4695) (-21.5505, 1.27, -180.8195) (-21.5505, 1.27, -187.1695) (-21.5505, 1.27, -193.5195) (-21.5505, 1.27, -199.8695) (-21.5505, 1.27, -206.2195) (-21.5505, 1.27, -212.5695) (-21.5505, 1.27, -218.9195) (-21.5505, 1.27, -225.2695) (-21.5505, 1.27, -231.6195) (-21.5505, 1.27, -237.9695) (-21.5505, 1.27, -244.3195) (-21.5505, 1.27, -250.6695) (-21.5505, 1.27, -257.0195) (-21.5505, 1.27, -263.3695) (-21.5505, 1.27, -269.7195) (-21.5505, 1.27, -276.0695) (-21.5505, 1.27, -282.4195) (-21.5505, 1.27, -288.7695) (-21.5505, 1.27, -295.1195) (-21.5505, 1.27, -301.4695) (-21.5505, 1.27, -307.8195) (-21.5505, 1.27, -314.1695) (-21.5505, 1.27, -320.5195) (-21.5505, 1.27, -326.8695) (-15.2005, 1.27, -34.7695) (-15.2005, 1.27, -41.1195) (-15.2005, 1.27, -47.4695) (-15.2005, 1.27, -53.8195) (-15.2005, 1.27, -60.1695) (-15.2005, 1.27, -66.5195) (-15.2005, 1.27, -72.8695) (-15.2005, 1.27, -79.2195) (-15.2005, 1.27, -85.5695) (-15.2005, 1.27, -91.9195) (-15.2005, 1.27, -98.2695) (-15.2005, 1.27, -104.6195) (-15.2005, 1.27, -110.9695) (-15.2005, 1.27, -117.3195) (-15.2005, 1.27, -149.0695) (-15.2005, 1.27, -155.4195) (-15.2005, 1.27, -161.7695) (-15.2005, 1.27, -168.1195) (-15.2005, 1.27, -174.4695) (-15.2005, 1.27, -180.8195) (-15.2005, 1.27, -187.1695) (-15.2005, 1.27, -193.5195) (-15.2005, 1.27, -199.8695) (-15.2005, 1.27, -206.2195) (-15.2005, 1.27, -212.5695) (-15.2005, 1.27, -218.9195) (-15.2005, 1.27, -225.2695) (-15.2005, 1.27, -231.6195) (-15.2005, 1.27, -237.9695) (-15.2005, 1.27, -244.3195) (-15.2005, 1.27, -250.6695) (-15.2005, 1.27, -257.0195) (-15.2005, 1.27, -263.3695) (-15.2005, 1.27, -269.7195) (-15.2005, 1.27, -276.0695) (-15.2005, 1.27, -282.4195) (-15.2005, 1.27, -288.7695) (-15.2005, 1.27, -295.1195) (-15.2005, 1.27, -301.4695) (-15.2005, 1.27, -307.8195) (-15.2005, 1.27, -314.1695) (-15.2005, 1.27, -320.5195) (-15.2005, 1.27, -326.8695) (-8.8505, 1.27, -15.7195) (-8.8505, 1.27, -22.0695) (-8.8505, 1.27, -28.4195) (-8.8505, 1.27, -34.7695) (-8.8505, 1.27, -41.1195) (-8.8505, 1.27, -47.4695) (-8.8505, 1.27, -53.8195) (-8.8505, 1.27, -60.1695) (-8.8505, 1.27, -66.5195) (-8.8505, 1.27, -72.8695) (-8.8505, 1.27, -79.2195) (-8.8505, 1.27, -85.5695) (-8.8505, 1.27, -91.9195) (-8.8505, 1.27, -98.2695) (-8.8505, 1.27, -104.6195) (-8.8505, 1.27, -110.9695) (-8.8505, 1.27, -117.3195) (-8.8505, 1.27, -123.6695) (-8.8505, 1.27, -130.0195) (-8.8505, 1.27, -136.3695) (-8.8505, 1.27, -142.7195) (-8.8505, 1.27, -149.0695) (-8.8505, 1.27, -155.4195) (-8.8505, 1.27, -161.7695) (-8.8505, 1.27, -168.1195) (-8.8505, 1.27, -174.4695) (-8.8505, 1.27, -180.8195) (-8.8505, 1.27, -187.1695) (-8.8505, 1.27, -193.5195) (-8.8505, 1.27, -199.8695) (-8.8505, 1.27, -206.2195) (-8.8505, 1.27, -212.5695) (-8.8505, 1.27, -218.9195) (-8.8505, 1.27, -225.2695) (-8.8505, 1.27, -231.6195) (-8.8505, 1.27, -237.9695) (-8.8505, 1.27, -244.3195) (-8.8505, 1.27, -250.6695) (-8.8505, 1.27, -257.0195) (-8.8505, 1.27, -263.3695) (-8.8505, 1.27, -269.7195) (-8.8505, 1.27, -276.0695) (-8.8505, 1.27, -282.4195) (-8.8505, 1.27, -288.7695) (-8.8505, 1.27, -295.1195) (-8.8505, 1.27, -301.4695) (-8.8505, 1.27, -307.8195) (-8.8505, 1.27, -320.5195) (-8.8505, 1.27, -314.1695)
fillet "Fillet1" radius 31.75 4 edges at (-76.2, 0.635, 25.4266) (0, 0.635, 25.4266) (-76.2, 0.635, -342.9) (0, 0.635, -342.9)
body "Solid1"
